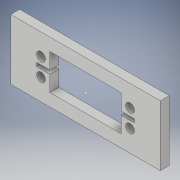
# Autodesk Inventor part: Cou-3
Saved by Autodesk Inventor 2018 (Build 220112000, 112)
## iProperties
Created: 2018-02-13
Part Number: Cou-3
Material: Generic
Document SubType Name: Modeling
Designer: Lilia
Density: 1 g/cm^3
Appearance: Default
Author: Lilia
Autodesk Inventor part; units mm, degrees
ref_plane "YZ Plane" through (0, 0, 0) normal (1, 0, 0) x (0, 1, 0)
ref_plane "XZ Plane" through (0, 0, 0) normal (0, 1, 0) x (-1, 0, 0)
ref_plane "XY Plane" through (0, 0, 0) normal (0, 0, 1) x (1, 0, 0)
sketch "Sketch1" plane through (0, 0, 0) normal (0, 0, 1) x (1, 0, 0)
  line L0 (-26, 13) -> (26, 13)
  line L1 (26, -13) -> (-26, -13)
  line L2 (-26, 13) -> (26, -13) construction
  line L3 (26, 13) -> (-26, -13) construction
  line L4 (-54.6, 22.1) -> (54.6, 22.1)
  line L5 (54.6, 22.1) -> (54.6, -22.1)
  line L6 (54.6, -22.1) -> (-54.6, -22.1)
  line L7 (-54.6, -22.1) -> (-54.6, 22.1)
  line L8 (-54.6, 22.1) -> (54.6, -22.1) construction
  line L9 (54.6, 22.1) -> (-54.6, -22.1) construction
  line L10 (-26, 1.3) -> (-35.75, 1.3)
  line L11 (-35.75, 1.3) -> (-35.75, -1.3)
  line L12 (-35.75, -1.3) -> (-26, -1.3)
  line L13 (26, 1.3) -> (35.75, 1.3)
  line L14 (35.75, 1.3) -> (35.75, -1.3)
  line L15 (35.75, -1.3) -> (26, -1.3)
  line L16 (-26, 1.3) -> (-26, 13)
  line L17 (-26, -13) -> (-26, -1.3)
  line L18 (26, -1.3) -> (26, -13)
  line L19 (26, 1.3) -> (26, 13)
  point P0 (0, 0)
  point P1 (-35.75, 0)
  point P2 (0, 0)
  dimension "CInt" = 52
  dimension "LInt" = 26
  dimension "Cext" = 109.2
  dimension "Lext" = 44.2
  dimension "Cpeq" = 9.75
  dimension "Lpeq" = 2.6
  dimension "d10" = 9.75
  dimension "d11" = 2.6
  constraints: 40 end point, 7 equal length, 6 midpoint, 4 horizontal, 3 perpendicular, 1 horizontal alignment, 1 point on line, 1 vertical
  measures "CInt" distance of L0.start L0.end
  measures "LInt" distance of L1.end L0.start
  measures "Cext" distance of L4.start L4.end
  measures "Lext" distance of L6.end L4.start
  measures "Cpeq" distance of L10.start L10.end
  measures "Lpeq" distance of L10.end L11.end
  measures "d10" distance of L13.start L13.end
  measures "d11" distance of L13.end L14.end
extrude "Extrusion1" add sketch "Sketch1" along normal mid plane 6.5
sketch "Sketch8" plane through (0, 0, 3.25) normal (0, 0, 1) x (1, 0, 0)
  point P0 (0, 0)
hole "Hole1" at (-32.5, 6.5, 3.25) direction (0, 0, -1) diameter 6.5 end through all
pattern_linear "Rectangular Pattern1" count 2 spacing 13 along (0, -1, 0) of "Hole1"
hole "Hole2" at (32.5, 6.6, 3.25) direction (0, 0, -1) diameter 6.5 end through all
pattern_linear "Rectangular Pattern2" count 2 spacing 13 along (0, -1, 0) of "Hole2"
body "Solid1"
